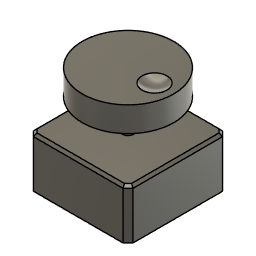
Knob Base  Basic v2 (Autodesk Fusion 360 design; units mm, degrees)
Autodesk Fusion 360 part; units mm, degrees
sketch "Sketch1" plane through (0, 0, 0) normal (0, 1, 0) x (1, 0, 0)
  line L0 (30, 30) -> (-30, 30)
  line L1 (-30, 30) -> (-30, -30)
  line L2 (-30, -30) -> (30, -30)
  line L3 (30, -30) -> (30, 30)
  line L4 (30, 30) -> (-30, -30) construction
  line L5 (-30, 30) -> (30, -30) construction
  circle A0 centre (0, 0) radius 3.5
  circle A1 centre (0, 0) radius 6.5
  line L6 (27, 27) -> (-27, 27)
  line L7 (-27, 27) -> (-27, -27)
  line L8 (-27, -27) -> (27, -27)
  line L9 (27, -27) -> (27, 27)
  line L10 (-16.3934, -27) -> (-27, -16.3934)
  line L11 (27, -16.3934) -> (16.3934, -27)
  line L12 (16.3934, 27) -> (27, 16.3934)
  line L13 (-27, 16.3934) -> (-16.3934, 27)
  dimension "d1" = 60
  dimension "d2" = 60
  dimension "d3" = 7
  dimension "d4" = 13
  dimension "d9" = -3
  dimension "d12" = 15
  dimension "d14" = 360
  constraint horizontal L0
  constraint perpendicular L0 L1
  constraint parallel L0 L2
  constraint parallel L1 L3
  constraint coincident L4 A0.centre
  constraint coincident L5 A0.centre
  constraint coincident A0.centre A1.centre
  constraint coincident L8 L10.start
  constraint coincident L7 L10.end
  constraint perpendicular L4 L10
  measures "d1" distance of L1.end L2.end
  measures "d2" distance of L0.end L1.end
  measures "d3" diameter of A0
  measures "d4" diameter of A1
  measures "d12" distance of L10.start L10.end
extrude "Extrude1" add sketch "Sketch1" along normal blind 2 contours L0 L1 L2 L3 | A1 | L6 L9 L12 | L6 L7 L8 L9 L10 L11 L12 L13 | L6 L7 L13 | L8 L9 L11 | L7 L8 L10 makes body 1
extrude "Extrude2" add sketch "Sketch1" against normal blind 5 contours A1 bodies 1
extrude "Extrude3" add sketch "Sketch1" against normal blind 28 contours L0 L1 L2 L3 bodies 1
extrude "Extrude4" add sketch "Sketch1" against normal blind 24 contours L6 L9 L12 | L6 L7 L13 | L8 L9 L11 | L7 L8 L10 bodies 1
sketch "Sketch2" plane through (0, -24, 0) normal (0, -1, 0) x (1, 0, 0)
  line L0 (-27, 16.3934) -> (-16.3934, 27)
  line L1 (-16.3934, 27) -> (-27, 27)
  line L2 (-27, 27) -> (-27, 16.3934)
  circle A0 centre (-23.818, 23.818) radius 1.5
  line L3 (-27, 27) -> (-21.6967, 21.6967) construction
  line L4 (-16.3934, 27) -> (-27, 16.3934)
  dimension "d17" = 3
  dimension "d23" = 4.5
  constraint coincident L1.end L2.start
  constraint midpoint L0 L3.end
  constraint coincident A0.centre L3
  measures "d17" diameter of A0
  measures "d23" distance of A0.centre L1.end
extrude "Extrude5" cut sketch "Sketch2" against normal blind 20 contours A0 bodies 1
pattern_circular "C-Pattern1" count 4 over 360 about axis through (0, 1.75, 0) along (0, 1, 0) of "Extrude5"
sketch "Sketch3" plane through (0, -28, 0) normal (0, -1, 0) x (1, 0, 0)
  line L0 (27, 27) -> (27, -27)
  line L1 (27, -27) -> (-27, -27)
  line L2 (-27, -27) -> (-27, 27)
  line L3 (-27, 27) -> (27, 27)
  line L4 (30, -30) -> (30, 30)
  line L5 (30, 30) -> (-30, 30)
  line L6 (-30, 30) -> (-30, -30)
  line L7 (-30, -30) -> (30, -30)
  line L8 (26.5, -26.5) -> (-26.5, -26.5)
  line L9 (-26.5, -26.5) -> (-26.5, 26.5)
  line L10 (-26.5, 26.5) -> (26.5, 26.5)
  line L11 (26.5, 26.5) -> (26.5, -26.5)
  line L12 (-26.5, -26.5) -> (26.5, 26.5) construction
  circle A0 centre (-23.818, -23.818) radius 1.6
  dimension "d24" = 0.5
  dimension "d30" = 3.2
  dimension "d31" = 4.5
  constraint coincident L12 A0.centre
  measures "d30" diameter of A0
  measures "d31" distance of L1.end A0.centre
extrude "Extrude6" add sketch "Sketch3" against normal blind 2 from surface at -2 separate body contours L8 L9 L10 L11 | A0 makes body 2
extrude "Extrude7" cut sketch "Sketch3" against normal blind 4 contours A0 bodies 2
pattern_circular "C-Pattern2" count 4 over 360 about axis through (0, 1.75, 0) along (0, 1, 0) of "Extrude7"
sketch "Sketch4" plane through (0, 0, -30) normal (0, 0, -1) x (-1, 0, 0)
  line L0 (30, -28) -> (30, 2)
  line L1 (30, 2) -> (-30, 2)
  line L2 (-30, 2) -> (-30, -28)
  line L3 (-30, -28) -> (30, -28)
  line L4 (-16, -6) -> (16, -6)
  line L5 (16, -6) -> (16, -18)
  line L6 (16, -18) -> (-16, -18)
  line L7 (-16, -18) -> (-16, -6)
  line L8 (-26.5, -28) -> (26.5, -28)
  dimension "d36" = 8
  dimension "d37" = 10
  dimension "d38" = 14
  dimension "d39" = 14
  constraint horizontal L4
  constraint vertical L5
  constraint horizontal L6
  constraint vertical L7
  measures "d36" distance of L1 L4
  measures "d37" distance of L6 L8
  measures "d38" distance of L2 L7
  measures "d39" distance of L0 L5
extrude "Extrude8" cut sketch "Sketch4" against normal blind 5 contours L4 L5 L6 L7 bodies 1
fillet "Fillet1" radius 5 4 edges at (-16, -18, -28.5) (-16, -6, -28.5) (16, -6, -28.5) (16, -18, -28.5) on bodies 1
chamfer "Chamfer1" distance 3 angle 45 4 edges at (30, -13, -30) (-30, -13, -30) (-30, -13, 30) (30, -13, 30) on bodies 1
chamfer "Chamfer2" distance 1.5 angle 45 8 edges at (0, 2, 30) (-28.5, 2, 28.5) (-30, 2, 0) (-28.5, 2, -28.5) (0, 2, -30) (28.5, 2, -28.5) (30, 2, 0) (28.5, 2, 28.5) on bodies 1
chamfer "Chamfer3" distance 0.75 angle 45 16 edges at (0, -18, -27) (-14.5355, -16.5355, -27) (-16, -12, -27) (-14.5355, -7.4645, -27) (0, -6, -27) (14.5355, -7.4645, -27) (16, -12, -27) (14.5355, -16.5355, -27) (0, -18, -30) (14.5355, -16.5355, -30) (16, -12, -30) (14.5355, -7.4645, -30) (0, -6, -30) (-14.5355, -7.4645, -30) (-16, -12, -30) (-14.5355, -16.5355, -30) on bodies 1
sketch "Sketch6" plane through (0, 0, 0) normal (0, 1, 0) x (1, 0, 0)
  circle A0 centre (0, 0) radius 27.5
  dimension "d48" = 55
  constraint coincident A0.centre origin
  measures "d48" diameter of A0
extrude "Extrude9" add sketch "Sketch6" along normal blind 15 from surface at 20 separate body makes body 3
sketch "Sketch7" plane through (0, 20, 0) normal (0, -1, 0) x (1, 0, 0)
  circle A0 centre (0, 0) radius 27.5
  circle A1 centre (0, 0) radius 3
  line L0 (-1.5, 2.5981) -> (-1.5, -2.5981)
  dimension "d53" = 6
  dimension "d54" = 1.5
  constraint concentric A0 A1
  constraint coincident A1 L0.start
  constraint coincident A1 L0.end
  constraint vertical L0
  measures "d53" diameter of A1
  measures "d54" distance of A0.centre L0
extrude "Extrude10" cut sketch "Sketch7" against normal blind 6 contours A1 L0 picked at (-0.6347, 0.9309) bodies 3
extrude "Extrude11" cut sketch "Sketch7" against normal blind 1 contours A1 L0 picked at (-1.7331, -0.6802) bodies 3
sketch "Sketch8" plane through (0, 0, 0) normal (0, 0, 1) x (1, 0, 0)
  circle A0 centre (16, 48) radius 15
  line L0 (27.5, 35) -> (-27.5, 35)
  line L1 (0, 35) -> (0, 85) construction
  line L2 (16, 35) -> (16, 85) construction
  line L3 (16, 33) -> (16, 63)
  dimension "d59" = 30
  dimension "d60" = 13
  dimension "d61" = 50
  dimension "d63" = 50
  dimension "d64" = 16
  constraint midpoint L0 L1.start
  constraint perpendicular L0 L1
  constraint coincident L0 L2.start
  constraint perpendicular L0 L2
  constraint coincident A0.centre L2
  constraint coincident A0 L3.start
  constraint coincident L2 L3.end
  constraint coincident A0 L3.end
  constraint perpendicular L0 L3
  measures "d59" diameter of A0
  measures "d60" distance of A0.centre L0
  measures "d61" distance of L1.start L1.end
  measures "d63" distance of L2.start L2.end
  measures "d64" distance of L1 L2
revolve "Revolve1" cut sketch "Sketch8" angle 360 about axis through (16, 35, 0) along (0, 1, 0) contours A0 L0 L3 | A0 L0 L3 picked at (16.7116, 53.6158) picked at (16.651, 33.7092) bodies 3
sketch "Sketch9" plane through (0, 35, 0) normal (0, 1, 0) x (-1, 0, 0)
  circle A0 centre (-16, 0) radius 7.4833
  circle A1 centre (0, 0) radius 27.5
  circle A2 centre (14.5, 0) radius 10.5
  line L0 (0, 0) -> (27.5, 0) construction
  circle A3 centre (0, 0) radius 3 construction
  dimension "d66" = 21
  dimension "d67" = 14.5
  dimension "d68" = 6
  constraint coincident A1.centre L0.start
  constraint coincident A1 L0.end
  constraint horizontal L0
  constraint coincident A2.centre L0
  measures "d66" diameter of A2
  measures "d67" distance of A2.centre A1.centre
  measures "d68" diameter of A3
extrude "Extrude12" cut sketch "Sketch9" against normal blind 9.5 from surface at -2 contours A2 bodies 3
pattern_circular "C-Pattern3" count 3 over 360 about axis through (0, 1.75, 0) along (0, 1, 0) of "Extrude12"
named bodies: "Knob Base Basic Main", "Knob Base Basic Cover", "Knob Base Basic Knob"
